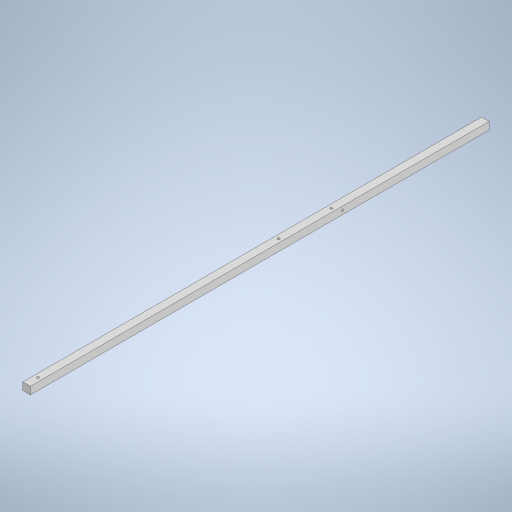
# Autodesk Inventor part: Dai
Saved by Autodesk Inventor 2023 (Build 270158000, 158)
## iProperties
Created: 2022-10-14
Part Number: Dai
Material: 一般
Document SubType Name: Modeling
Designer: banru
Density: 1 g/cm^3
Appearance: 既定
Author: banru
Autodesk Inventor part; units mm, degrees
ref_plane "YZ Plane" through (0, 0, 0) normal (1, 0, 0) x (0, 1, 0)
ref_plane "XZ Plane" through (0, 0, 0) normal (0, 1, 0) x (-1, 0, 0)
ref_plane "XY Plane" through (0, 0, 0) normal (0, 0, 1) x (1, 0, 0)
sketch "スケッチ1" plane through (0, 0, 0) normal (0, 1, 0) x (-1, 0, 0)
  line L0 (0, 0) -> (10, 0)
  line L1 (10, 0) -> (10, -610)
  line L2 (10, -610) -> (0, -610)
  line L3 (0, -610) -> (0, 0)
  dimension "d0" = 10
  dimension "d1" = 610
  constraints: 8 end point, 2 parallel, 1 horizontal, 1 perpendicular
  measures "d0" distance of L1.end L2.end
  measures "d1" distance of L0.end L1.end
extrude "押し出し1" add sketch "スケッチ1" along normal blind 10
sketch "スケッチ2" plane through (0, 10, 0) normal (0, 1, 0) x (1, 0, 0)
  line L0 (-10, 0) -> (0, 0) projected
  point P0 (-5, 405)
  point P1 (-5, 0)
  point P2 (-5, 0)
  dimension "d4" = 405
  constraints: 2 midpoint, 1 vertical alignment
  measures "d4" distance of point (-5, 0) point (-5, 405)
hole "穴1" at (-5, 10, -405) direction (0, -1, 0) diameter 3.1 end through all
sketch "スケッチ3" plane through (0, 0, 0) normal (1, 0, 0) x (0, 0, -1)
  line L0 (0, 0) -> (0, 10) projected
  point P0 (415, 5)
  point P1 (0, 5)
  point P2 (0, 5)
  dimension "d12" = 415
  constraints: 2 midpoint, 1 horizontal alignment
  measures "d12" distance of point (0, 5) point (415, 5)
hole "穴2" at (0, 5, -415) direction (-1, 0, 0) diameter 3.1 end through all
sketch "スケッチ4" plane through (0, 10, 0) normal (0, 1, 0) x (1, 0, 0)
  line L0 (-10, 0) -> (0, 0) projected
  point P0 (-5, 15)
  point P1 (-5, 335)
  point P2 (-5, 0)
  point P3 (-5, 0)
  point P4 (-5, 0)
  point P5 (-5, 0)
  dimension "d20" = 15
  dimension "d21" = 335
  constraints: 4 midpoint, 2 vertical alignment
  measures "d20" distance of point (-5, 0) point (-5, 15)
  measures "d21" distance of point (-5, 0) point (-5, 335)
hole "穴3" at (-5, 10, -15) at (-5, 10, -335) direction (0, -1, 0) diameter 3.1 end through all
